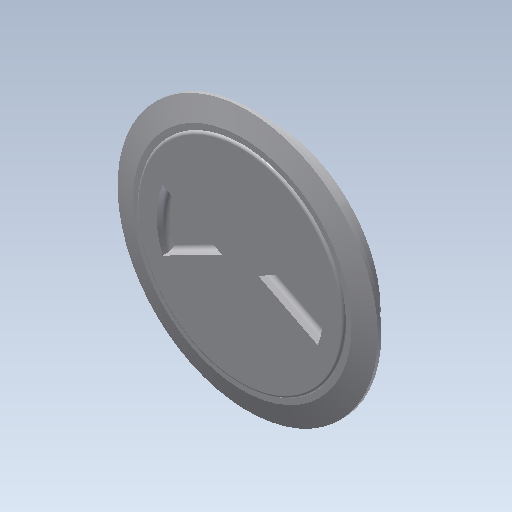
# Autodesk Inventor part: hatch
Saved by Autodesk Inventor 2020 (Build 240168000, 168)
## iProperties
Created: 2016-11-10
Part Number: hatch
Material: Generic
Document SubType Name: Modeling
Designer: jous
Density: 1 g/cm^3
Appearance: Default
Mass: 200.606 g
Surface Area: 736.731 cm^2
Volume: 200.606 cm^3
Author: jous
Autodesk Inventor part; units mm, degrees
ref_plane "YZ Plane" through (0, 0, 0) normal (1, 0, 0) x (0, 1, 0)
ref_plane "XZ Plane" through (0, 0, 0) normal (0, 1, 0) x (-1, 0, 0)
ref_plane "XY Plane" through (0, 0, 0) normal (0, 0, 1) x (1, 0, 0)
sketch "Sketch1" plane through (0, 0, 0) normal (0, 0, 1) x (1, 0, 0)
  circle A0 centre (0, 0) radius 94
  circle A1 centre (0, 0) radius 75
  line L0 (-13, 0) -> (-56, 22)
  line L1 (-130, 0) -> (137, 0) construction
  line L2 (0, 131.4545) -> (0, -117) construction
  line L3 (-13, 0) -> (-56, -22)
  line L4 (0, -131.4545) -> (0, 117) construction
  arc A2 (-56, 22) -> (-56, -22) centre (0, 0) ccw
  line L5 (13, 0) -> (56, 22)
  line L6 (13, 0) -> (56, -22)
  arc A3 (56, -22) -> (56, 22) centre (0, 0) ccw
  circle A4 centre (0, 0) radius 78.5
  dimension "d0" = 188
  dimension "d6" = 150
  dimension "d16" = 157
  constraints: 14 end point, 6 symmetric about line, 5 centre point, 4 point on circle, 3 coincident, 1 concentric, 1 horizontal, 1 perpendicular, 1 other
  measures "d0" diameter of A0
  measures "d6" diameter of A1
  measures "d16" diameter of A4
extrude "Extrusion1" add sketch "Sketch1" along normal blind 6.5 contours A0 | A4
extrude "Extrusion3" add sketch "Sketch1" along normal blind 8 contours A1
fillet "Fillet2" radius 2 1 edges at (-75, 0, 8)
chamfer "Chamfer1" distance 15 angle 15 1 edges at (-94, 0, 6.5) measured on face at (-71.1692, 50.8207, 6.5)
extrude "Extrusion4" add sketch "Sketch1" along normal blind 1 contours L3 A2 L0 | L5 A3 L6
fillet "Fillet3" radius 3 6 edges at (-60.1664, 0, 1) (-34.5, 11, 1) (-34.5, -11, 1) (34.5, 11, 1) (34.5, -11, 1) (60.1664, 0, 1)
extrude "Extrusion5" add sketch "Sketch1" against normal blind 15 contours A4
body "Solid1"
